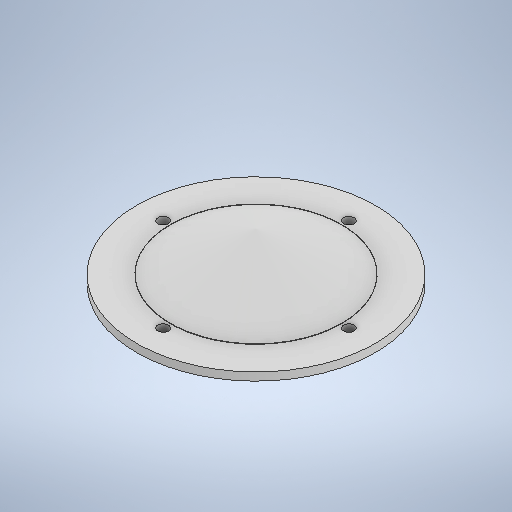
# Autodesk Inventor part: tarcza
Saved by Autodesk Inventor 2025 (Build 290162000, 162)
## iProperties
Created: 2024-12-31
Part Number: tarcza
Material: Ogólny
Document SubType Name: Modeling
Designer: Laptop
Density: 1 g/cm^3
Appearance: Domyślna
Author: Laptop
Autodesk Inventor part; units mm, degrees
ref_plane "YZ Plane" through (0, 0, 0) normal (1, 0, 0) x (0, 1, 0)
ref_plane "XZ Plane" through (0, 0, 0) normal (0, 1, 0) x (-1, 0, 0)
ref_plane "XY Plane" through (0, 0, 0) normal (0, 0, 1) x (1, 0, 0)
sketch "Szkic1" plane through (0, 0, 0) normal (0, 1, 0) x (-1, 0, 0)
  circle A0 centre (0, 0) radius 45
  circle A1 centre (35, 0) radius 1.5
  circle A2 centre (-35, 0) radius 1.5
  circle A3 centre (0, 35) radius 1.5
  circle A4 centre (0, -35) radius 1.5
  dimension "d0" = 90
  dimension "d30" = 3
  dimension "d31" = 3
  dimension "d32" = 3
  dimension "d33" = 3
  constraints: 5 centre point, 1 coincident
  measures "d0" diameter of A0
  measures "d30" diameter of A1
  measures "d31" diameter of A2
  measures "d32" diameter of A3
  measures "d33" diameter of A4
extrude "Wyciągnięcie proste1" add sketch "Szkic1" along normal blind 3 contours A0 | A1 | A2 | A3 | A4
sketch "Szkic4" plane through (0, 0, 0) normal (0, -1, 0) x (1, 0, 0)
  circle A0 centre (0, 0) radius 2.5 projected
  circle A1 centre (0, 0) radius 5
  dimension "d19" = 10
  constraints: 1 centre point, 1 coincident
  measures "d19" diameter of A1
extrude "Wyciągnięcie proste5" cut sketch "Szkic4" against normal blind 2 contours A0 | A1
sketch "Szkic8" plane through (0, 2, 0) normal (0, -1, 0) x (1, 0, 0)
  point P0 (0, 0)
sketch "Szkic17" plane through (0, 3, 0) normal (0, 1, 0) x (1, 0, 0)
  circle A0 centre (-35, 0) radius 2
  circle A1 centre (0, 35) radius 2
  circle A2 centre (0, -35) radius 2
  circle A3 centre (35, 0) radius 2
  point P0 (0, 0)
  dimension "d34" = 4
  dimension "d35" = 4
  dimension "d36" = 4
  dimension "d37" = 4
  constraints: 4 centre point
  measures "d34" diameter of A0
  measures "d35" diameter of A1
  measures "d36" diameter of A2
  measures "d37" diameter of A3
extrude "Wyciągnięcie proste9" cut sketch "Szkic17" against normal blind 47
sketch "Szkic19" plane through (0, 3, 0) normal (0, 1, 0) x (1, 0, 0)
  point P0 (0, 0)
sketch "Szkic20" plane through (0, 3, 0) normal (0, 1, 0) x (1, 0, 0)
  circle A0 centre (0, 0) radius 5 projected
  circle A1 centre (0, 0) radius 32.25
  dimension "d47" = 64.5
  constraints: 1 centre point, 1 coincident
  measures "d47" diameter of A1
extrude "Wyciągnięcie proste11" add sketch "Szkic20" along normal blind 15 contours A0 | A1
chamfer "Faza1" distance 32.25 angle 24.7 1 edges at (-32.25, 18, 0) measured on face at (15.449, 18, -8.9531)
